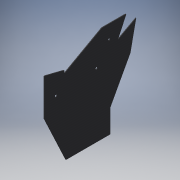
# Autodesk Inventor part: end_plate
Saved by Autodesk Inventor 2018.2 (Build 222227000, 227)
## iProperties
Created: 2017-10-22
Part Number: end_plate
Material: 木材 (オーク)
Document SubType Name: Modeling
Designer: ku_sk
Density: 0.76 g/cm^3
Appearance: カーボンファイバー
Mass: 1235.6 g
Surface Area: 6637.57 cm^2
Volume: 1625.78 cm^3
Author: ku_sk
Autodesk Inventor part; units mm, degrees
ref_plane "YZ Plane" through (0, 0, 0) normal (1, 0, 0) x (0, 1, 0)
ref_plane "XZ Plane" through (0, 0, 0) normal (0, 1, 0) x (-1, 0, 0)
ref_plane "XY Plane" through (0, 0, 0) normal (0, 0, 1) x (1, 0, 0)
sketch "スケッチ1" plane through (0, 0, 0) normal (1, 0, 0) x (0, 1, 0)
  line L0 (-670, 192.9198) -> (-670, 500)
  line L1 (-670, 500) -> (-350, 650)
  line L2 (-350, 650) -> (-90, 650)
  line L3 (0, 250) -> (0, 0)
  line L4 (-124.5856, 512.0252) -> (-145.1979, 512.0252)
  line L5 (-145.1979, 512.0252) -> (0, 250)
  line L6 (-90, 650) -> (-124.5856, 512.0252)
  line L7 (-249.1712, 52.2397) -> (-510, 192.9198)
  line L8 (-510, 192.9198) -> (-670, 192.9198)
  line L9 (0, 0) -> (-249.1712, 52.2397)
  dimension "d2" = 150
  dimension "d3" = 320
  dimension "d4" = 250
  dimension "d5" = 670
  dimension "d79" = 260
  constraints: 20 end point, 3 horizontal, 1 coincident, 1 parallel, 1 perpendicular
  measures "d2" distance from line of L0.end L2
  measures "d3" distance from line of L1.end L0
  measures "d4" distance of L3.start L3.end
  measures "d5" distance between parallel lines of L0 L3
  measures "d79" distance of L1.end L2.end
extrude "押し出し1" add sketch "スケッチ1" along normal blind 5
sketch "スケッチ8" plane through (5, 0, 0) normal (1, 0, 0) x (0, 0, -1)
  circle A0 centre (-570, -250) radius 7.5
  circle A1 centre (-288.2903, -224.7089) radius 7.5
  line L0 (0, 0) -> (-250, 0) projected
  line L1 (-570, -250) -> (-290.3837, -264.6541)
  line L2 (-290.3837, -264.6541) -> (-288.2903, -224.7089)
  line L3 (0, -804) -> (0, 134) projected
  dimension "d65" = 15
  dimension "d66" = 15
  dimension "d77" = 250
  dimension "d88" = 40
  dimension "d89" = 280
  dimension "d90" = 3
  dimension "d91" = 570
  constraints: 4 end point, 2 centre point, 1 coincident, 1 perpendicular
  measures "d65" diameter of A0
  measures "d66" diameter of A1
  measures "d77" distance from line of L0 L1.start
  measures "d88" distance of L1.end L2.end
  measures "d89" distance of L1.start L1.end
  measures "d90" angle of L0 L1
  measures "d91" distance from line of L3 L1.start
extrude "押し出し8" cut sketch "スケッチ8" against normal through all
sketch "スケッチ12" plane through (5, 0, 0) normal (1, 0, 0) x (0, 0, -1)
  circle A0 centre (-200, -95) radius 6.6799
  point P0 (0, 0)
  dimension "d84" = 200
  dimension "d85" = 95
  constraints: 1 centre point
  measures "d84" horizontal distance of point (0, 0) A0.centre
  measures "d85" vertical distance of point (0, 0) A0.centre
extrude "押し出し11" cut sketch "スケッチ12" against normal through all
sketch "スケッチ13" plane through (5, 0, 0) normal (1, 0, 0) x (0, 0, -1)
  line L0 (0, -804) -> (0, 134) projected
  line L1 (130, 0) -> (-780, 0) projected
  line L2 (-80, 0) -> (-121.7476, -89.528)
  line L3 (-121.7476, -89.528) -> (-1.0516, -5.0157)
  line L4 (-52.2397, -249.1712) -> (0, 0) projected
  dimension "d95" = 80
  dimension "d96" = 115
  dimension "d97" = 30
  constraints: 4 end point, 2 point on line
  measures "d95" distance from line of L0 L2.start
  measures "d96" angle of L1 L2
  measures "d97" angle of L3 L2
extrude "押し出し12" cut sketch "スケッチ13" against normal through all
fillet "フィレット2" radius 3 6 edges at (2.5, -89.528, 121.7476) (2.5, -5.0157, 1.0516) (2.5, 0, 80) (2.5, -145.1979, 512.0252) (2.5, -124.5856, 512.0252) (2.5, -90, 650)
sketch "スケッチ14" plane through (5, 0, 0) normal (1, 0, 0) x (0, 0, -1)
  line L0 (-117.0159, -79.3808) -> (-81.9901, -4.2679) projected
  line L1 (-52.2397, -249.1712) -> (-2.608, -12.4393) projected
  line L2 (-7.2648, -9.3663) -> (-112.5762, -83.1061) projected
  line L3 (-81.9901, -4.2679) -> (-139.0675, -126.6706)
  line L4 (-139.0675, -126.6706) -> (-12.3616, -58.9618)
  line L5 (-52.2397, -249.1712) -> (-2.608, -12.4393) projected
  line L6 (-12.3616, -58.9618) -> (-2.608, -12.4393)
  line L7 (-2.608, -12.4393) -> (0, 0)
  line L8 (0, 0) -> (-81.9901, -4.2679)
  constraints: 10 end point, 3 collinear, 1 point on line
extrude "押し出し13" cut sketch "スケッチ14" against normal through all
